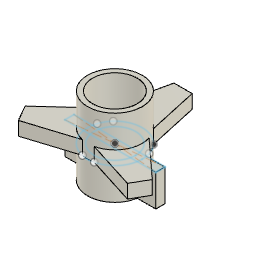
接着剤スタンド (Autodesk Fusion 360 design; units mm, degrees)
Autodesk Fusion 360 part; units mm, degrees
note: some values were not read from the file. Set by a fixed rule: which sketch regions a step uses.
sketch "スケッチ1" plane through (0, 0, 0) normal (0, 0, 1) x (1, 0, 0)
  circle A0 centre (0, 0) radius 4.9
  circle A1 centre (0, 0) radius 6
  line L0 (-2, 15) -> (2, 15)
  line L1 (2, 15) -> (4.4261, 4.0509)
  line L2 (0, 15) -> (0, 11)
  line L3 (-2, 15) -> (-4.4261, 4.0509)
  line L4 (-13.9904, -5.7679) -> (-5.7212, 1.8076)
  line L5 (-11.9904, -9.2321) -> (-13.9904, -5.7679)
  line L6 (-11.9904, -9.2321) -> (-1.2952, -5.8585)
  line L7 (11.9904, -9.2321) -> (1.2952, -5.8585)
  line L8 (13.9904, -5.7679) -> (11.9904, -9.2321)
  line L9 (13.9904, -5.7679) -> (5.7212, 1.8076)
  dimension "d1" = 9.8
  dimension "d2" = 12
  dimension "d4" = 360
  constraint coincident A0.centre A1.centre
  constraint horizontal L0
  constraint coincident A1 L1.end
  constraint midpoint L0 L2.start
  constraint perpendicular L0 L2
  constraint symmetric L0.end L2 L0.start
  constraint symmetric L1.end L2 L3.end
  measures "d1" diameter of A0
  measures "d2" diameter of A1
extrude "押し出し1" add sketch "スケッチ1" along normal blind 2 contours A0 | A1 | A1 L7 L8 L9 | A1 L0 L1 L3 | A1 L4 L5 L6 makes body 1
extrude "押し出し2" add sketch "スケッチ1" along normal blind 8 from surface at 2 contours A1 bodies 1
move_face "面を移動1" by (0, 0, 1) 3 faces at (10.3743, -6.0305, 2) (-10.3923, -6, 2) (0, 12, 2) on bodies 1
sketch "スケッチ2" plane through (0, 0, 0) normal (0, 0, 1) x (1, 0, 0)
  circle A0 centre (0, 0) radius 6
  circle A1 centre (0, 0) radius 4.55
  line L0 (10, -1) -> (-10, -1)
  line L1 (-10, -1) -> (-10, 1)
  line L2 (-10, 1) -> (10, 1)
  line L3 (10, 1) -> (10, -1)
  line L4 (10, -1) -> (-10, 1) construction
  line L5 (-10, -1) -> (10, 1) construction
  point P0 (4.4261, 4.0509)
  point P1 (5.7212, 1.8076)
  point P2 (-5.7212, 1.8076)
  point P3 (-1.2952, -5.8585)
  point P4 (1.2952, -5.8585)
  point P5 (-4.4261, 4.0509)
  dimension "d10" = 9.1
  dimension "d11" = 12
  dimension "d12" = 20
  constraint coincident A0.centre A1.centre
  constraint coincident P0 A0
  constraint horizontal L0
  constraint perpendicular L0 L1
  constraint parallel L0 L2
  constraint parallel L1 L3
  constraint coincident L4 A0.centre
  constraint coincident L5 A0.centre
  measures "d10" diameter of A1
  measures "d11" diameter of A0
  measures "d12" distance of L1.end L2.end
extrude "押し出し3" add sketch "スケッチ2" against normal blind 7 separate body contours A0 A1 L0 L2 | A0 L0 L2 L3 | A0 A1 L2 | A0 A1 L0 | A0 A1 L0 L2 | A0 L0 L1 L2 makes body 2
chamfer "面取り1" distance 0.5 angle 45 1 edges at (-4.2421, -1.6454, -7) on bodies 2
chamfer "面取り2" distance 0.5 angle 45 1 edges at (-4.2421, 1.6454, 0) on bodies 2
named bodies: "stand", "cap"
